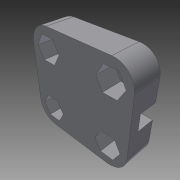
# Autodesk Inventor part: bottom
Saved by Autodesk Inventor 2014 (Build 180170000, 170)
## iProperties
Created: 2016-03-14
Part Number: bottom
Material: Generic
Document SubType Name: Modeling
Designer: buben
Density: 1 g/cm^3
Appearance: Default
Author: buben
Autodesk Inventor part; units mm, degrees
ref_plane "YZ Plane" through (0, 0, 0) normal (1, 0, 0) x (0, 1, 0)
ref_plane "XZ Plane" through (0, 0, 0) normal (0, 1, 0) x (-1, 0, 0)
ref_plane "XY Plane" through (0, 0, 0) normal (0, 0, 1) x (1, 0, 0)
sketch "Sketch1" plane through (0, 0, 0) normal (0, 1, 0) x (-1, 0, 0)
  line L0 (0, 0) -> (-32, 0)
  line L1 (-32, 0) -> (-32, -30)
  line L2 (-32, -30) -> (0, -30)
  line L3 (0, -30) -> (0, 0)
  dimension "d0" = 30
  dimension "d1" = 32
  constraints: 8 end point, 2 parallel, 1 horizontal, 1 perpendicular
  measures "d0" distance of L2.end L0.start
  measures "d1" distance of L0.start L0.end
extrude "Extrusion1" add sketch "Sketch1" along normal blind 3
sketch "Sketch2" plane through (0, 3, 0) normal (0, 1, 0) x (1, 0, 0)
  line L0 (0, 0) -> (32, 0) projected
  line L1 (32, 0) -> (32, 30) projected
  line L2 (32, 30) -> (0, 30) projected
  line L3 (0, 30) -> (0, 0) projected
  line L4 (9.25, 20.5) -> (22.75, 20.5)
  line L5 (22.75, 20.5) -> (22.75, 9.5)
  line L6 (22.75, 9.5) -> (9.25, 9.5)
  line L7 (9.25, 9.5) -> (9.25, 20.5)
  point P0 (9.25, 15)
  point P1 (0, 15)
  point P2 (16, 9.5)
  point P3 (16, 0)
  dimension "d4" = 11
  dimension "d5" = 13.5
  constraints: 8 end point, 4 midpoint, 2 parallel, 1 horizontal, 1 horizontal alignment, 1 perpendicular, 1 vertical alignment
  measures "d4" distance of L6.end L4.start
  measures "d5" distance of L5.end L6.end
extrude "Extrusion2" add sketch "Sketch2" along normal blind 5.5
sketch "Sketch3" plane through (0, 8.5, 0) normal (0, 1, 0) x (1, 0, 0)
  line L0 (22.75, 20.5) -> (22.75, 9.5) projected
  line L1 (32, 0) -> (32, 30) projected
  line L2 (22.75, 17.5) -> (32, 17.5)
  line L3 (32, 17.5) -> (32, 12.5)
  line L4 (32, 12.5) -> (22.75, 12.5)
  line L5 (22.75, 12.5) -> (22.75, 17.5)
  point P0 (22.75, 15)
  point P1 (22.75, 15)
  dimension "d8" = 5
  constraints: 8 end point, 2 midpoint, 2 parallel, 2 point on line, 1 coincident, 1 horizontal, 1 perpendicular
  measures "d8" distance of L4.end L2.start
extrude "Extrusion3" cut sketch "Sketch3" against normal up to surface (5.5 mm away)
sketch "Sketch4" plane through (0, 8.5, 0) normal (0, 1, 0) x (1, 0, 0)
  line L0 (32, 30) -> (0, 30) projected
  line L1 (0, 30) -> (0, 0) projected
  line L2 (6, 24) -> (26, 24) construction
  line L3 (26, 24) -> (26, 6) construction
  line L4 (26, 6) -> (6, 6) construction
  line L5 (6, 6) -> (6, 24) construction
  circle A0 centre (6, 24) radius 2
  circle A1 centre (6, 6) radius 2
  circle A2 centre (26, 6) radius 2
  circle A3 centre (26, 24) radius 2
  point P0 (6, 15)
  point P1 (0, 15)
  point P2 (16, 24)
  point P3 (16, 30)
  dimension "d11" = 4
  dimension "d18" = 18
  dimension "d19" = 20
  constraints: 8 end point, 4 centre point, 4 coincident, 4 midpoint, 3 equal radius, 2 parallel, 1 horizontal, 1 horizontal alignment, 1 perpendicular, 1 vertical alignment
  measures "d11" diameter of A0
  measures "d18" distance of L4.end L2.start
  measures "d19" distance of L2.start L2.end
extrude "Extrusion4" cut sketch "Sketch4" against normal through all
fillet "Fillet1" radius 6 4 edges at (0, 4.25, -30) (0, 4.25, 0) (32, 4.25, 0) (32, 4.25, -30)
sketch "Sketch5" plane through (0, 0, 0) normal (0, -1, 0) x (1, 0, 0)
  circle A0 centre (26, -6) radius 2 projected
  circle A1 centre (6, -24) radius 2 projected
  circle A2 centre (6, -6) radius 2 projected
  circle A3 centre (26, -24) radius 2 projected
  line L0 (3.9793, -9.5) -> (1.9585, -6)
  line L1 (1.9585, -6) -> (3.9793, -2.5)
  line L2 (3.9793, -2.5) -> (8.0207, -2.5)
  line L3 (8.0207, -2.5) -> (10.0415, -6)
  line L4 (10.0415, -6) -> (8.0207, -9.5)
  line L5 (8.0207, -9.5) -> (3.9793, -9.5)
  line L6 (8.0207, -20.5) -> (10.0415, -24)
  line L7 (10.0415, -24) -> (8.0207, -27.5)
  line L8 (8.0207, -27.5) -> (3.9793, -27.5)
  line L9 (3.9793, -27.5) -> (1.9585, -24)
  line L10 (1.9585, -24) -> (3.9793, -20.5)
  line L11 (3.9793, -20.5) -> (8.0207, -20.5)
  line L12 (21.9585, -24) -> (23.9793, -20.5)
  line L13 (23.9793, -20.5) -> (28.0207, -20.5)
  line L14 (28.0207, -20.5) -> (30.0415, -24)
  line L15 (30.0415, -24) -> (28.0207, -27.5)
  line L16 (28.0207, -27.5) -> (23.9793, -27.5)
  line L17 (23.9793, -27.5) -> (21.9585, -24)
  line L18 (21.9585, -6) -> (23.9793, -2.5)
  line L19 (23.9793, -2.5) -> (28.0207, -2.5)
  line L20 (28.0207, -2.5) -> (30.0415, -6)
  line L21 (30.0415, -6) -> (28.0207, -9.5)
  line L22 (28.0207, -9.5) -> (23.9793, -9.5)
  line L23 (23.9793, -9.5) -> (21.9585, -6)
  point P0 (0, 0)
  point P1 (6, -27.5)
  dimension "d21" = 7
  constraints: 48 end point, 4 coincident, 4 horizontal, 3 equal length, 1 midpoint, 52 other
  measures "d21" distance between parallel lines of L1 L4
extrude "Extrusion5" cut sketch "Sketch5" against normal blind 6
body "Solid1"
